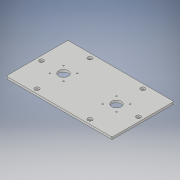
# Autodesk Inventor part: BT001_trajan20_21
Saved by Autodesk Inventor 2022.2 (Build 262287000, 287)
## iProperties
Company: HTBLA Kaindorf
RuleStatus: InUse
Created: 2022-08-03
Part Number: BT001_trajan20_21
Project: Zeichenmaschine_v2
Material: Generisch
Description: Platte Stepper Motoren
Document SubType Name: Modeling
Designer: trajan20
Density: 1 g/cm^3
Appearance: Vorgabe
Mass: 161.904 g
Surface Area: 709.746 cm^2
Volume: 161.904 cm^3
AfterDocNew0: iProperties-Editor_aufrufen
Author: jan
Keywords: 2021
Autodesk Inventor part; units mm, degrees
ref_plane "YZ Plane" through (0, 0, 0) normal (1, 0, 0) x (0, 1, 0)
ref_plane "XZ Plane" through (0, 0, 0) normal (0, 1, 0) x (-1, 0, 0)
sketch "Skizze3" plane through (0, 0, 0) normal (0, 0, 1) x (1, 0, 0)
  line L0 (0, 0) -> (-140, 0)
  line L1 (-140, 0) -> (-140, 120)
  line L2 (-140, 240) -> (0, 240)
  line L3 (0, 240) -> (0, 0)
  line L4 (-34.5565, 44.5) -> (-109.2584, 44.5) construction
  line L5 (-42.5521, 75.5) -> (-110.6291, 75.5) construction
  line L6 (-85.5, 104.3529) -> (-85.5, 36.2759) construction
  line L7 (-54.5, 102.2969) -> (-54.5, 32.1639) construction
  line L8 (-70, -15.9958) -> (-70, 12.0858) construction
  circle A0 centre (-70, 60) radius 11
  circle A1 centre (-85.5, 75.5) radius 1.5
  circle A2 centre (-85.5, 44.5) radius 1.5
  circle A3 centre (-54.5, 44.5) radius 1.5
  circle A4 centre (-54.5, 75.5) radius 1.5
  line L9 (-140, 120) -> (0, 120) construction
  line L10 (-140, 120) -> (-140, 240)
  line L11 (-148.6913, 60) -> (9.8942, 60) construction
  line L12 (-160.7703, 180) -> (-4.1331, 180) construction
  point P0 (-70, 0)
  point P1 (-70, 10)
  point P2 (-130, 60)
  point P3 (-140, 180)
  point P4 (-140, 60)
  point P5 (-130, 180)
  point P6 (-10, 180)
  point P7 (-10, 60)
  point P8 (-70, 230)
  dimension "d4" = 240
  dimension "d5" = 140
  dimension "d6" = 31
  dimension "d7" = 31
  dimension "d8" = 15.5
  dimension "d9" = 15.5
  dimension "d10" = 60
  dimension "d11" = 22
  dimension "d12" = 3
  dimension "d13" = 3
  dimension "d14" = 3
  dimension "d15" = 3
  dimension "d22" = 10
  dimension "d23" = 10
  dimension "d24" = 10
  dimension "d25" = 10
  dimension "d26" = 10
  dimension "d34" = 10
  constraints: 26 end point, 18 point on line, 5 centre point, 5 coincident, 4 horizontal, 4 midpoint, 4 perpendicular, 3 parallel, 3 vertical
  measures "d4" distance between parallel lines of L2 L0
  measures "d5" distance between parallel lines of L1 L3
  measures "d6" distance between parallel lines of L6 L7
  measures "d7" distance between parallel lines of L5 L4
  measures "d8" distance from line of L7 point (-70, 60)
  measures "d9" distance from line of L5 point (-70, 60)
  measures "d10" distance from line of L0 point (-70, 60)
  measures "d11" diameter of A0
  measures "d12" diameter of A3
  measures "d13" diameter of A2
  measures "d14" diameter of A4
  measures "d15" diameter of A1
  measures "d22" distance from line of L0 point (-70, 10)
  measures "d23" distance from line of point (-10, 60) L3
  measures "d24" distance from line of L3 point (-10, 180)
  measures "d25" distance from line of L10 point (-130, 180)
  measures "d26" distance from line of L1 point (-130, 60)
  measures "d34" distance from line of L2 point (-70, 230)
extrude "Extrusion3" add sketch "Skizze3" against normal blind 5 contours L0 L1 L10 L2 L3 | A0 | A1 | A2 | A3 | A4
fillet "Rundung1" radius 2 4 edges at (0, 0, -2.5) (0, 240, -2.5) (-140, 240, -2.5) (-140, 0, -2.5)
ref_plane "Arbeitsebene1" through (-140, 120, 0) normal (0, 1, 0) x (1, 0, 0)
extrude "Extrusion4" cut sketch "Skizze3" against normal through all contours A0 | A1 | A2 | A3 | A4
mirror "Spiegeln1" about plane through (-140, 120, 0) normal (0, 1, 0) of "Extrusion4"
hole "Bohrung1" at (-70, 60, 0) at (-70, 10, 0) at (-130, 60, 0) at (-130, 180, 0) at (-10, 180, 0) at (-10, 60, 0) at (-70, 230, 0) direction (0, 0, -1) diameter 5.5 end through all counterbore diameter 10 counterbore depth 3.9
equation "\"d8\" = 0.5 * d6"
equation "\"d9\" = d8"
equation "\"d23\" = d22"
equation "\"d24\" = d23"
equation "\"d25\" = d22"
equation "\"d26\" = d25"
